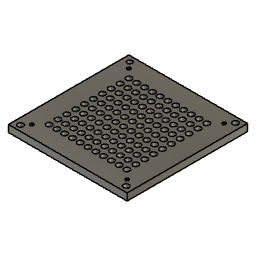
WC_Zwischenboden (Autodesk Fusion 360 design; units mm, degrees)
Autodesk Fusion 360 part; units mm, degrees
note: some values were not read from the file. Set by a fixed rule: which face or edge a step refers to.
(part 1 of 3)
sketch "Skizze1" plane through (0, 0, 0) normal (0, 0, 1) x (1, 0, 0)
  line L0 (0.1074, 0.221) -> (507.9074, 0.221)
  line L1 (507.9074, 0.221) -> (507.9074, -514.979)
  line L2 (507.9074, -514.979) -> (0.1074, -514.979)
  line L3 (0.1074, -514.979) -> (0.1074, 0.221)
  circle A0 centre (87.5074, -86.379) radius 12
  circle A1 centre (28.1074, -23.779) radius 10.8095
  circle A2 centre (479.9074, -23.779) radius 12
  circle A3 centre (120.8074, -86.379) radius 12
  circle A4 centre (154.1074, -86.379) radius 12
  circle A5 centre (187.4074, -86.379) radius 12
  circle A6 centre (220.7074, -86.379) radius 12
  circle A7 centre (254.0074, -86.379) radius 12
  circle A8 centre (287.3074, -86.379) radius 12
  circle A9 centre (320.6074, -86.379) radius 12
  circle A10 centre (353.9074, -86.379) radius 12
  circle A11 centre (387.2074, -86.379) radius 12
  circle A12 centre (420.5074, -86.379) radius 12
  circle A13 centre (87.5074, -124.379) radius 12
  circle A14 centre (120.8074, -124.379) radius 12
  circle A15 centre (154.1074, -124.379) radius 12
  circle A16 centre (187.4074, -124.379) radius 12
  circle A17 centre (220.7074, -124.379) radius 12
  circle A18 centre (254.0074, -124.379) radius 12
  circle A19 centre (287.3074, -124.379) radius 12
  circle A20 centre (320.6074, -124.379) radius 12
  circle A21 centre (353.9074, -124.379) radius 12
  circle A22 centre (387.2074, -124.379) radius 12
  circle A23 centre (420.5074, -124.379) radius 12
  circle A24 centre (87.5074, -162.379) radius 12
  circle A25 centre (120.8074, -162.379) radius 12
  circle A26 centre (154.1074, -162.379) radius 12
  circle A27 centre (187.4074, -162.379) radius 12
  circle A28 centre (220.7074, -162.379) radius 12
  circle A29 centre (254.0074, -162.379) radius 12
  circle A30 centre (287.3074, -162.379) radius 12
  circle A31 centre (320.6074, -162.379) radius 12
  circle A32 centre (353.9074, -162.379) radius 12
  circle A33 centre (387.2074, -162.379) radius 12
  circle A34 centre (420.5074, -162.379) radius 12
  circle A35 centre (87.5074, -200.379) radius 12
  circle A36 centre (120.8074, -200.379) radius 12
  circle A37 centre (154.1074, -200.379) radius 12
  circle A38 centre (187.4074, -200.379) radius 12
  circle A39 centre (220.7074, -200.379) radius 12
  circle A40 centre (254.0074, -200.379) radius 12
  circle A41 centre (287.3074, -200.379) radius 12
  circle A42 centre (320.6074, -200.379) radius 12
  circle A43 centre (353.9074, -200.379) radius 12
  circle A44 centre (387.2074, -200.379) radius 12
  circle A45 centre (420.5074, -200.379) radius 12
  circle A46 centre (87.5074, -238.379) radius 12
  circle A47 centre (120.8074, -238.379) radius 12
  circle A48 centre (154.1074, -238.379) radius 12
  circle A49 centre (187.4074, -238.379) radius 12
  circle A50 centre (220.7074, -238.379) radius 12
  circle A51 centre (254.0074, -238.379) radius 12
  circle A52 centre (287.3074, -238.379) radius 12
  circle A53 centre (320.6074, -238.379) radius 12
  circle A54 centre (353.9074, -238.379) radius 12
  circle A55 centre (387.2074, -238.379) radius 12
  circle A56 centre (420.5074, -238.379) radius 12
  circle A57 centre (87.5074, -276.379) radius 12
  circle A58 centre (120.8074, -276.379) radius 12
  circle A59 centre (154.1074, -276.379) radius 12
  circle A60 centre (187.4074, -276.379) radius 12
  circle A61 centre (220.7074, -276.379) radius 12
  circle A62 centre (254.0074, -276.379) radius 12
  circle A63 centre (287.3074, -276.379) radius 12
  circle A64 centre (320.6074, -276.379) radius 12
  circle A65 centre (353.9074, -276.379) radius 12
  circle A66 centre (387.2074, -276.379) radius 12
  circle A67 centre (420.5074, -276.379) radius 12
  circle A68 centre (87.5074, -314.379) radius 12
  circle A69 centre (120.8074, -314.379) radius 12
  circle A70 centre (154.1074, -314.379) radius 12
  circle A71 centre (187.4074, -314.379) radius 12
  circle A72 centre (220.7074, -314.379) radius 12
  circle A73 centre (254.0074, -314.379) radius 12
  circle A74 centre (287.3074, -314.379) radius 12
  circle A75 centre (320.6074, -314.379) radius 12
  circle A76 centre (353.9074, -314.379) radius 12
  circle A77 centre (387.2074, -314.379) radius 12
  circle A78 centre (420.5074, -314.379) radius 12
  circle A79 centre (87.5074, -352.379) radius 12
  circle A80 centre (120.8074, -352.379) radius 12
  circle A81 centre (154.1074, -352.379) radius 12
  circle A82 centre (187.4074, -352.379) radius 12
  circle A83 centre (220.7074, -352.379) radius 12
  circle A84 centre (254.0074, -352.379) radius 12
  circle A85 centre (287.3074, -352.379) radius 12
  circle A86 centre (320.6074, -352.379) radius 12
  circle A87 centre (353.9074, -352.379) radius 12
  circle A88 centre (387.2074, -352.379) radius 12
  circle A89 centre (420.5074, -352.379) radius 12
  circle A90 centre (87.5074, -390.379) radius 12
  circle A91 centre (120.8074, -390.379) radius 12
  circle A92 centre (154.1074, -390.379) radius 12
  circle A93 centre (187.4074, -390.379) radius 12
  circle A94 centre (220.7074, -390.379) radius 12
  circle A95 centre (254.0074, -390.379) radius 12
  circle A96 centre (287.3074, -390.379) radius 12
  circle A97 centre (320.6074, -390.379) radius 12
  circle A98 centre (353.9074, -390.379) radius 12
  circle A99 centre (387.2074, -390.379) radius 12
  circle A100 centre (420.5074, -390.379) radius 12
  circle A101 centre (87.5074, -428.379) radius 12
  circle A102 centre (120.8074, -428.379) radius 12
  circle A103 centre (154.1074, -428.379) radius 12
  circle A104 centre (187.4074, -428.379) radius 12
  circle A105 centre (220.7074, -428.379) radius 12
  circle A106 centre (254.0074, -428.379) radius 12
  circle A107 centre (287.3074, -428.379) radius 12
  circle A108 centre (320.6074, -428.379) radius 12
  circle A109 centre (353.9074, -428.379) radius 12
  circle A110 centre (387.2074, -428.379) radius 12
  circle A111 centre (420.5074, -428.379) radius 12
  circle A112 centre (28.1074, -490.979) radius 12
  circle A113 centre (479.9074, -490.979) radius 12
  dimension "d1" = 24
  dimension "d2" = 87.4
  dimension "d3" = 86.6
  dimension "d6" = 21.619
  dimension "d7" = 28
  dimension "d8" = 24
  dimension "d38" = 24
  dimension "d39" = 24
  dimension "d40" = 28
  dimension "d131" = 33.3
  dimension "d132" = -38
  dimension "d133" = 38
  dimension "d134" = 38
  dimension "d135" = 38
  dimension "d136" = 38
  dimension "d137" = 38
  dimension "d138" = 38
  dimension "d139" = 38
  dimension "d140" = 38
  dimension "d141" = 38
  dimension "d142" = 86.6
  dimension "d143" = 33.3
  dimension "d144" = 33.3
  dimension "d145" = 33.3
  dimension "d146" = 33.3
  dimension "d147" = 33.3
  dimension "d148" = 33.3
  dimension "d149" = 33.3
  dimension "d150" = 33.3
  dimension "d151" = 33.3
  dimension "d152" = 33.3
  dimension "d153" = 87.4
  dimension "d154" = 24
  dimension "d155" = 28
  dimension "d156" = 24
  dimension "d157" = 24
  dimension "d158" = 24
  dimension "d159" = 28
  constraint horizontal L0
  constraint vertical L1
  constraint vertical L3
  measures "d1" diameter of A0
  measures "d2" distance of L3 A0.centre
  measures "d3" distance of L0 A0.centre
  measures "d6" diameter of A1
  measures "d7" distance of L3 A1.centre
  measures "d8" distance of L0 A1.centre
  measures "d38" diameter of A2
  measures "d39" distance of L0 A2.centre
  measures "d40" distance of L1 A2.centre
  measures "d133" distance of A0.centre A13.centre
  measures "d134" distance of A13.centre A24.centre
  measures "d135" distance of A24.centre A35.centre
  measures "d136" distance of A35.centre A46.centre
  measures "d137" distance of A46.centre A57.centre
  measures "d138" distance of A57.centre A68.centre
  measures "d139" distance of A68.centre A79.centre
  measures "d140" distance of A79.centre A90.centre
  measures "d141" distance of A90.centre A101.centre
  measures "d142" distance of L2 A101.centre
  measures "d143" distance of A0.centre A3.centre
  measures "d144" distance of A3.centre A4.centre
  measures "d145" distance of A4.centre A5.centre
  measures "d146" distance of A5.centre A6.centre
  measures "d147" distance of A6.centre A7.centre
  measures "d148" distance of A7.centre A8.centre
  measures "d149" distance of A8.centre A9.centre
  measures "d150" distance of A9.centre A10.centre
  measures "d151" distance of A10.centre A11.centre
  measures "d152" distance of A11.centre A12.centre
  measures "d153" distance of L1 A12.centre
  measures "d154" diameter of A112
  measures "d155" distance of L3 A112.centre
  measures "d156" distance of L2 A112.centre
  measures "d157" diameter of A113
  measures "d158" distance of L2 A113.centre
  measures "d159" distance of L1 A113.centre
extrude "Extrusion1" add sketch "Skizze1" along normal blind 20
sketch "Skizze2" plane through (0, 0, 20) normal (0, 0, 1) x (-1, 0, 0)
  circle A0 centre (-387.2074, 124.379) radius 12
  circle A1 centre (-353.9074, 124.379) radius 12
  circle A2 centre (-320.6074, 124.379) radius 12
  circle A3 centre (-287.3074, 124.379) radius 12
  circle A4 centre (-254.0074, 124.379) radius 12
  circle A5 centre (-220.7074, 124.379) radius 12
  circle A6 centre (-187.4074, 124.379) radius 12
  circle A7 centre (-154.1074, 124.379) radius 12
  circle A8 centre (-120.8074, 124.379) radius 12
  circle A9 centre (-87.5074, 124.379) radius 12
  circle A10 centre (-420.5074, 86.379) radius 12
  circle A11 centre (-387.2074, 86.379) radius 12
  circle A12 centre (-353.9074, 86.379) radius 12
  circle A13 centre (-320.6074, 86.379) radius 12
  circle A14 centre (-287.3074, 86.379) radius 12
  circle A15 centre (-254.0074, 86.379) radius 12
  circle A16 centre (-220.7074, 86.379) radius 12
  circle A17 centre (-187.4074, 86.379) radius 12
  circle A18 centre (-154.1074, 86.379) radius 12
  circle A19 centre (-120.8074, 86.379) radius 12
  circle A20 centre (-479.9074, 23.779) radius 12
  circle A21 centre (-28.1074, 23.779) radius 10.8095
  circle A22 centre (-87.5074, 86.379) radius 12
  circle A23 centre (-387.2074, 238.379) radius 12
  circle A24 centre (-420.5074, 238.379) radius 12
  circle A25 centre (-87.5074, 276.379) radius 12
  circle A26 centre (-120.8074, 276.379) radius 12
  circle A27 centre (-154.1074, 276.379) radius 12
  circle A28 centre (-187.4074, 276.379) radius 12
  circle A29 centre (-220.7074, 276.379) radius 12
  circle A30 centre (-254.0074, 276.379) radius 12
  circle A31 centre (-287.3074, 276.379) radius 12
  circle A32 centre (-320.6074, 276.379) radius 12
  circle A33 centre (-353.9074, 276.379) radius 12
  circle A34 centre (-387.2074, 276.379) radius 12
  circle A35 centre (-420.5074, 276.379) radius 12
  circle A36 centre (-87.5074, 314.379) radius 12
  circle A37 centre (-120.8074, 314.379) radius 12
  circle A38 centre (-154.1074, 314.379) radius 12
  circle A39 centre (-187.4074, 314.379) radius 12
  circle A40 centre (-220.7074, 314.379) radius 12
  circle A41 centre (-254.0074, 314.379) radius 12
  circle A42 centre (-287.3074, 314.379) radius 12
  circle A43 centre (-320.6074, 314.379) radius 12
  circle A44 centre (-353.9074, 314.379) radius 12
  circle A45 centre (-387.2074, 314.379) radius 12
  circle A46 centre (-420.5074, 314.379) radius 12
  circle A47 centre (-87.5074, 352.379) radius 12
  circle A48 centre (-120.8074, 352.379) radius 12
  circle A49 centre (-154.1074, 352.379) radius 12
  circle A50 centre (-187.4074, 352.379) radius 12
  circle A51 centre (-220.7074, 352.379) radius 12
  circle A52 centre (-254.0074, 352.379) radius 12
  circle A53 centre (-353.9074, 238.379) radius 12
  circle A54 centre (-320.6074, 238.379) radius 12
  circle A55 centre (-287.3074, 238.379) radius 12
  circle A56 centre (-254.0074, 238.379) radius 12
  circle A57 centre (-220.7074, 238.379) radius 12
  circle A58 centre (-187.4074, 238.379) radius 12
  circle A59 centre (-154.1074, 238.379) radius 12
  circle A60 centre (-120.8074, 238.379) radius 12
  circle A61 centre (-87.5074, 238.379) radius 12
  circle A62 centre (-420.5074, 200.379) radius 12
  circle A63 centre (-387.2074, 200.379) radius 12
  circle A64 centre (-353.9074, 200.379) radius 12
  circle A65 centre (-320.6074, 200.379) radius 12
  circle A66 centre (-287.3074, 200.379) radius 12
  circle A67 centre (-254.0074, 200.379) radius 12
  circle A68 centre (-220.7074, 200.379) radius 12
  circle A69 centre (-187.4074, 200.379) radius 12
  circle A70 centre (-154.1074, 200.379) radius 12
  circle A71 centre (-120.8074, 200.379) radius 12
  circle A72 centre (-87.5074, 200.379) radius 12
  circle A73 centre (-420.5074, 162.379) radius 12
  circle A74 centre (-387.2074, 162.379) radius 12
  circle A75 centre (-353.9074, 162.379) radius 12
  circle A76 centre (-320.6074, 162.379) radius 12
  circle A77 centre (-287.3074, 162.379) radius 12
  circle A78 centre (-254.0074, 162.379) radius 12
  circle A79 centre (-220.7074, 162.379) radius 12
  circle A80 centre (-187.4074, 162.379) radius 12
  circle A81 centre (-154.1074, 162.379) radius 12
  circle A82 centre (-120.8074, 162.379) radius 12
  circle A83 centre (-87.5074, 162.379) radius 12
  circle A84 centre (-420.5074, 124.379) radius 12
  circle A85 centre (-320.6074, 352.379) radius 12
  circle A86 centre (-353.9074, 352.379) radius 12
  circle A87 centre (-387.2074, 352.379) radius 12
  circle A88 centre (-420.5074, 352.379) radius 12
  circle A89 centre (-87.5074, 390.379) radius 12
  circle A90 centre (-120.8074, 390.379) radius 12
  circle A91 centre (-154.1074, 390.379) radius 12
  circle A92 centre (-187.4074, 390.379) radius 12
  circle A93 centre (-220.7074, 390.379) radius 12
  circle A94 centre (-254.0074, 390.379) radius 12
  circle A95 centre (-287.3074, 390.379) radius 12
  circle A96 centre (-320.6074, 390.379) radius 12
  circle A97 centre (-353.9074, 390.379) radius 12
  circle A98 centre (-387.2074, 390.379) radius 12
  circle A99 centre (-420.5074, 390.379) radius 12
  circle A100 centre (-87.5074, 428.379) radius 12
  circle A101 centre (-120.8074, 428.379) radius 12
  circle A102 centre (-154.1074, 428.379) radius 12
  circle A103 centre (-187.4074, 428.379) radius 12
  circle A104 centre (-220.7074, 428.379) radius 12
  circle A105 centre (-254.0074, 428.379) radius 12
  circle A106 centre (-287.3074, 428.379) radius 12
  circle A107 centre (-320.6074, 428.379) radius 12
  circle A108 centre (-353.9074, 428.379) radius 12
  circle A109 centre (-387.2074, 428.379) radius 12
  circle A110 centre (-420.5074, 428.379) radius 12
  circle A111 centre (-28.1074, 490.979) radius 12
  circle A112 centre (-479.9074, 490.979) radius 12
  circle A113 centre (-287.3074, 352.379) radius 12
  line L0 (-0.1074, 514.979) -> (-507.9074, 514.979)
  line L1 (-507.9074, 514.979) -> (-507.9074, -0.221)
  line L2 (-507.9074, -0.221) -> (-0.1074, -0.221)
  line L3 (-0.1074, -0.221) -> (-0.1074, 514.979)
extrude "Extrusion2" add sketch "Skizze2" along normal blind 10
sketch "Skizze4" plane through (0, 0, 0) normal (0, 0, -1) x (1, 0, 0)
  circle A0 centre (387.2074, 124.379) radius 12
  circle A1 centre (353.9074, 124.379) radius 12
  circle A2 centre (320.6074, 124.379) radius 12
  circle A3 centre (287.3074, 124.379) radius 12
  circle A4 centre (254.0074, 124.379) radius 12
  circle A5 centre (220.7074, 124.379) radius 12
  circle A6 centre (187.4074, 124.379) radius 12
  circle A7 centre (154.1074, 124.379) radius 12
  circle A8 centre (120.8074, 124.379) radius 12
  circle A9 centre (87.5074, 124.379) radius 12
  circle A10 centre (420.5074, 86.379) radius 12
  circle A11 centre (387.2074, 86.379) radius 12
  circle A12 centre (353.9074, 86.379) radius 12
  circle A13 centre (320.6074, 86.379) radius 12
  circle A14 centre (287.3074, 86.379) radius 12
  circle A15 centre (254.0074, 86.379) radius 12
  circle A16 centre (220.7074, 86.379) radius 12
  circle A17 centre (187.4074, 86.379) radius 12
  circle A18 centre (154.1074, 86.379) radius 12
  circle A19 centre (120.8074, 86.379) radius 12
  circle A20 centre (479.9074, 23.779) radius 12
  circle A21 centre (28.1074, 23.779) radius 10.8095
  circle A22 centre (87.5074, 86.379) radius 12
  circle A23 centre (387.2074, 238.379) radius 12
  circle A24 centre (420.5074, 238.379) radius 12
  circle A25 centre (87.5074, 276.379) radius 12
  circle A26 centre (120.8074, 276.379) radius 12
  circle A27 centre (154.1074, 276.379) radius 12
  circle A28 centre (187.4074, 276.379) radius 12
  circle A29 centre (220.7074, 276.379) radius 12
  circle A30 centre (254.0074, 276.379) radius 12
  circle A31 centre (287.3074, 276.379) radius 12
  circle A32 centre (320.6074, 276.379) radius 12
  circle A33 centre (353.9074, 276.379) radius 12
  circle A34 centre (387.2074, 276.379) radius 12
  circle A35 centre (420.5074, 276.379) radius 12
  circle A36 centre (87.5074, 314.379) radius 12
  circle A37 centre (120.8074, 314.379) radius 12
  circle A38 centre (154.1074, 314.379) radius 12
  circle A39 centre (187.4074, 314.379) radius 12
  circle A40 centre (220.7074, 314.379) radius 12
  circle A41 centre (254.0074, 314.379) radius 12
  circle A42 centre (287.3074, 314.379) radius 12
  circle A43 centre (320.6074, 314.379) radius 12
  circle A44 centre (353.9074, 314.379) radius 12
  circle A45 centre (387.2074, 314.379) radius 12
  circle A46 centre (420.5074, 314.379) radius 12
  circle A47 centre (87.5074, 352.379) radius 12
  circle A48 centre (120.8074, 352.379) radius 12
  circle A49 centre (154.1074, 352.379) radius 12
  circle A50 centre (187.4074, 352.379) radius 12
  circle A51 centre (220.7074, 352.379) radius 12
  circle A52 centre (254.0074, 352.379) radius 12
  circle A53 centre (353.9074, 238.379) radius 12
  circle A54 centre (320.6074, 238.379) radius 12
  circle A55 centre (287.3074, 238.379) radius 12
  circle A56 centre (254.0074, 238.379) radius 12
  circle A57 centre (220.7074, 238.379) radius 12
  circle A58 centre (187.4074, 238.379) radius 12
  circle A59 centre (154.1074, 238.379) radius 12
  circle A60 centre (120.8074, 238.379) radius 12
  circle A61 centre (87.5074, 238.379) radius 12
  circle A62 centre (420.5074, 200.379) radius 12
  circle A63 centre (387.2074, 200.379) radius 12
  circle A64 centre (353.9074, 200.379) radius 12
  circle A65 centre (320.6074, 200.379) radius 12
  circle A66 centre (287.3074, 200.379) radius 12
  circle A67 centre (254.0074, 200.379) radius 12
  circle A68 centre (220.7074, 200.379) radius 12
  circle A69 centre (187.4074, 200.379) radius 12
  circle A70 centre (154.1074, 200.379) radius 12
  circle A71 centre (120.8074, 200.379) radius 12
  circle A72 centre (87.5074, 200.379) radius 12
  circle A73 centre (420.5074, 162.379) radius 12
  circle A74 centre (387.2074, 162.379) radius 12
  circle A75 centre (353.9074, 162.379) radius 12
  circle A76 centre (320.6074, 162.379) radius 12
  circle A77 centre (287.3074, 162.379) radius 12
  circle A78 centre (254.0074, 162.379) radius 12
  circle A79 centre (220.7074, 162.379) radius 12
  circle A80 centre (187.4074, 162.379) radius 12
  circle A81 centre (154.1074, 162.379) radius 12
  circle A82 centre (120.8074, 162.379) radius 12
  circle A83 centre (87.5074, 162.379) radius 12
  circle A84 centre (420.5074, 124.379) radius 12
  circle A85 centre (320.6074, 352.379) radius 12
  circle A86 centre (353.9074, 352.379) radius 12
  circle A87 centre (387.2074, 352.379) radius 12
  circle A88 centre (420.5074, 352.379) radius 12
  circle A89 centre (87.5074, 390.379) radius 12
  circle A90 centre (120.8074, 390.379) radius 12
  circle A91 centre (154.1074, 390.379) radius 12
  circle A92 centre (187.4074, 390.379) radius 12
  circle A93 centre (220.7074, 390.379) radius 12
  circle A94 centre (254.0074, 390.379) radius 12
  circle A95 centre (287.3074, 390.379) radius 12
  circle A96 centre (320.6074, 390.379) radius 12
  circle A97 centre (353.9074, 390.379) radius 12
  circle A98 centre (387.2074, 390.379) radius 12
  circle A99 centre (420.5074, 390.379) radius 12
  circle A100 centre (87.5074, 428.379) radius 12
  circle A101 centre (120.8074, 428.379) radius 12
  circle A102 centre (154.1074, 428.379) radius 12
  circle A103 centre (187.4074, 428.379) radius 12
  circle A104 centre (220.7074, 428.379) radius 12
  circle A105 centre (254.0074, 428.379) radius 12
  circle A106 centre (287.3074, 428.379) radius 12
  circle A107 centre (320.6074, 428.379) radius 12
  circle A108 centre (353.9074, 428.379) radius 12
  circle A109 centre (387.2074, 428.379) radius 12
  circle A110 centre (420.5074, 428.379) radius 12
  circle A111 centre (28.1074, 490.979) radius 12
  circle A112 centre (479.9074, 490.979) radius 12
  circle A113 centre (287.3074, 352.379) radius 12
  line L0 (507.9074, 514.979) -> (0.1074, 514.979)
  line L1 (0.1074, 514.979) -> (0.1074, -0.221)
  line L2 (0.1074, -0.221) -> (507.9074, -0.221)
  line L3 (507.9074, -0.221) -> (507.9074, 514.979)
  line L4 (10.1074, 464.979) -> (60.1074, 464.979)
  line L5 (60.1074, 464.979) -> (60.1074, 49.779)
  line L6 (60.1074, 49.779) -> (10.1074, 49.779)
  line L7 (10.1074, 49.779) -> (10.1074, 464.979)
  dimension "d180" = 50
  dimension "d181" = 50
  dimension "d182" = 10
  dimension "d183" = 50
  constraint horizontal L4
  constraint vertical L5
  constraint horizontal L6
  constraint vertical L7
  measures "d180" distance of L0 L4
  measures "d181" distance of L2 L6
  measures "d182" distance of L1 L7
  measures "d183" distance of L5 L7
extrude "Extrusion3" cut sketch "Skizze4" against normal blind 20 contours L4 L5 L6 L7
sketch "Skizze5" plane through (0, 0, 0) normal (0, 0, -1) x (1, 0, 0)
  line L0 (60.1074, 464.979) -> (60.1074, 49.779)
  line L1 (60.1074, 49.779) -> (10.1074, 49.779)
  line L2 (10.1074, 49.779) -> (10.1074, 464.979)
  line L3 (10.1074, 464.979) -> (60.1074, 464.979)
  circle A0 centre (387.2074, 124.379) radius 12
  circle A1 centre (353.9074, 124.379) radius 12
  circle A2 centre (320.6074, 124.379) radius 12
  circle A3 centre (287.3074, 124.379) radius 12
  circle A4 centre (254.0074, 124.379) radius 12
  circle A5 centre (220.7074, 124.379) radius 12
  circle A6 centre (187.4074, 124.379) radius 12
  circle A7 centre (154.1074, 124.379) radius 12
  circle A8 centre (120.8074, 124.379) radius 12
  circle A9 centre (87.5074, 124.379) radius 12
  circle A10 centre (420.5074, 86.379) radius 12
  circle A11 centre (387.2074, 86.379) radius 12
  circle A12 centre (353.9074, 86.379) radius 12
  circle A13 centre (320.6074, 86.379) radius 12
  circle A14 centre (287.3074, 86.379) radius 12
  circle A15 centre (254.0074, 86.379) radius 12
  circle A16 centre (220.7074, 86.379) radius 12
  circle A17 centre (187.4074, 86.379) radius 12
  circle A18 centre (154.1074, 86.379) radius 12
  circle A19 centre (120.8074, 86.379) radius 12
  circle A20 centre (479.9074, 23.779) radius 12
  circle A21 centre (28.1074, 23.779) radius 10.8095
  circle A22 centre (87.5074, 86.379) radius 12
  circle A23 centre (387.2074, 238.379) radius 12
  circle A24 centre (420.5074, 238.379) radius 12
  circle A25 centre (87.5074, 276.379) radius 12
  circle A26 centre (120.8074, 276.379) radius 12
  circle A27 centre (154.1074, 276.379) radius 12
  circle A28 centre (187.4074, 276.379) radius 12
  circle A29 centre (220.7074, 276.379) radius 12
  circle A30 centre (254.0074, 276.379) radius 12
  circle A31 centre (287.3074, 276.379) radius 12
  circle A32 centre (320.6074, 276.379) radius 12
  circle A33 centre (353.9074, 276.379) radius 12
  circle A34 centre (387.2074, 276.379) radius 12
  circle A35 centre (420.5074, 276.379) radius 12
  circle A36 centre (87.5074, 314.379) radius 12
  circle A37 centre (120.8074, 314.379) radius 12
  circle A38 centre (154.1074, 314.379) radius 12
  circle A39 centre (187.4074, 314.379) radius 12
  circle A40 centre (220.7074, 314.379) radius 12
  circle A41 centre (254.0074, 314.379) radius 12
  circle A42 centre (287.3074, 314.379) radius 12
  circle A43 centre (320.6074, 314.379) radius 12
  circle A44 centre (353.9074, 314.379) radius 12
  circle A45 centre (387.2074, 314.379) radius 12
  circle A46 centre (420.5074, 314.379) radius 12
  circle A47 centre (87.5074, 352.379) radius 12
  circle A48 centre (120.8074, 352.379) radius 12
  circle A49 centre (154.1074, 352.379) radius 12
  circle A50 centre (187.4074, 352.379) radius 12
  circle A51 centre (220.7074, 352.379) radius 12
  circle A52 centre (254.0074, 352.379) radius 12
  circle A53 centre (353.9074, 238.379) radius 12
  circle A54 centre (320.6074, 238.379) radius 12
  circle A55 centre (287.3074, 238.379) radius 12
  circle A56 centre (254.0074, 238.379) radius 12
  circle A57 centre (220.7074, 238.379) radius 12
  circle A58 centre (187.4074, 238.379) radius 12
  circle A59 centre (154.1074, 238.379) radius 12
  circle A60 centre (120.8074, 238.379) radius 12
  circle A61 centre (87.5074, 238.379) radius 12
  circle A62 centre (420.5074, 200.379) radius 12
  circle A63 centre (387.2074, 200.379) radius 12
  circle A64 centre (353.9074, 200.379) radius 12
  circle A65 centre (320.6074, 200.379) radius 12
  circle A66 centre (287.3074, 200.379) radius 12
  circle A67 centre (254.0074, 200.379) radius 12
  circle A68 centre (220.7074, 200.379) radius 12
  circle A69 centre (187.4074, 200.379) radius 12
  circle A70 centre (154.1074, 200.379) radius 12
  circle A71 centre (120.8074, 200.379) radius 12
  circle A72 centre (87.5074, 200.379) radius 12
  circle A73 centre (420.5074, 162.379) radius 12
  circle A74 centre (387.2074, 162.379) radius 12
  circle A75 centre (353.9074, 162.379) radius 12
  circle A76 centre (320.6074, 162.379) radius 12
  circle A77 centre (287.3074, 162.379) radius 12
  circle A78 centre (254.0074, 162.379) radius 12
  circle A79 centre (220.7074, 162.379) radius 12
  circle A80 centre (187.4074, 162.379) radius 12
  circle A81 centre (154.1074, 162.379) radius 12
  circle A82 centre (120.8074, 162.379) radius 12
  circle A83 centre (87.5074, 162.379) radius 12
  circle A84 centre (420.5074, 124.379) radius 12
  circle A85 centre (320.6074, 352.379) radius 12
  circle A86 centre (353.9074, 352.379) radius 12
  circle A87 centre (387.2074, 352.379) radius 12
  circle A88 centre (420.5074, 352.379) radius 12
  circle A89 centre (87.5074, 390.379) radius 12
  circle A90 centre (120.8074, 390.379) radius 12
  circle A91 centre (154.1074, 390.379) radius 12
  circle A92 centre (187.4074, 390.379) radius 12
  circle A93 centre (220.7074, 390.379) radius 12
  circle A94 centre (254.0074, 390.379) radius 12
  circle A95 centre (287.3074, 390.379) radius 12
  circle A96 centre (320.6074, 390.379) radius 12
  circle A97 centre (353.9074, 390.379) radius 12
  circle A98 centre (387.2074, 390.379) radius 12
  circle A99 centre (420.5074, 390.379) radius 12
  circle A100 centre (87.5074, 428.379) radius 12
  circle A101 centre (120.8074, 428.379) radius 12
  circle A102 centre (154.1074, 428.379) radius 12
  circle A103 centre (187.4074, 428.379) radius 12
  circle A104 centre (220.7074, 428.379) radius 12
  circle A105 centre (254.0074, 428.379) radius 12
  circle A106 centre (287.3074, 428.379) radius 12
  circle A107 centre (320.6074, 428.379) radius 12
  circle A108 centre (353.9074, 428.379) radius 12
  circle A109 centre (387.2074, 428.379) radius 12
  circle A110 centre (420.5074, 428.379) radius 12
  circle A111 centre (28.1074, 490.979) radius 12
  circle A112 centre (479.9074, 490.979) radius 12
  circle A113 centre (287.3074, 352.379) radius 12
  line L4 (507.9074, 514.979) -> (0.1074, 514.979)
  line L5 (0.1074, 514.979) -> (0.1074, -0.221)
  line L6 (0.1074, -0.221) -> (507.9074, -0.221)
  line L7 (507.9074, -0.221) -> (507.9074, 514.979)
  line L8 (50.1074, 504.979) -> (457.9074, 504.979)
  line L9 (457.9074, 504.979) -> (457.9074, 449.979)
  line L10 (457.9074, 449.979) -> (50.1074, 449.979)
  line L11 (50.1074, 449.979) -> (50.1074, 504.979)
  dimension "d186" = 50
  dimension "d187" = 50
  dimension "d188" = 10
  dimension "d189" = 55
  constraint horizontal L8
  constraint vertical L9
  constraint horizontal L10
  constraint vertical L11
  measures "d186" distance of L5 L11
  measures "d187" distance of L7 L9
  measures "d188" distance of L4 L8
  measures "d189" distance of L8 L10
extrude "Extrusion4" cut sketch "Skizze5" against normal blind 20 contours L0 L3 L8 L9 L10 L11
sketch "Skizze6" plane through (0, 0, 0) normal (0, 0, -1) x (1, 0, 0)
  line L0 (457.9074, 449.979) -> (60.1074, 449.979)
  line L1 (60.1074, 449.979) -> (60.1074, 49.779)
  line L2 (60.1074, 49.779) -> (10.1074, 49.779)
  line L3 (10.1074, 49.779) -> (10.1074, 464.979)
  line L4 (10.1074, 464.979) -> (50.1074, 464.979)
  line L5 (50.1074, 464.979) -> (50.1074, 504.979)
  line L6 (50.1074, 504.979) -> (457.9074, 504.979)
  line L7 (457.9074, 504.979) -> (457.9074, 449.979)
  circle A0 centre (387.2074, 124.379) radius 12
  circle A1 centre (353.9074, 124.379) radius 12
  circle A2 centre (320.6074, 124.379) radius 12
  circle A3 centre (287.3074, 124.379) radius 12
  circle A4 centre (254.0074, 124.379) radius 12
  circle A5 centre (220.7074, 124.379) radius 12
  circle A6 centre (187.4074, 124.379) radius 12
  circle A7 centre (154.1074, 124.379) radius 12
  circle A8 centre (120.8074, 124.379) radius 12
  circle A9 centre (87.5074, 124.379) radius 12
  circle A10 centre (420.5074, 86.379) radius 12
  circle A11 centre (387.2074, 86.379) radius 12
  circle A12 centre (353.9074, 86.379) radius 12
  circle A13 centre (320.6074, 86.379) radius 12
  circle A14 centre (287.3074, 86.379) radius 12
  circle A15 centre (254.0074, 86.379) radius 12
  circle A16 centre (220.7074, 86.379) radius 12
  circle A17 centre (187.4074, 86.379) radius 12
  circle A18 centre (154.1074, 86.379) radius 12
  circle A19 centre (120.8074, 86.379) radius 12
  circle A20 centre (479.9074, 23.779) radius 12
  circle A21 centre (28.1074, 23.779) radius 10.8095
  circle A22 centre (87.5074, 86.379) radius 12
  circle A23 centre (387.2074, 238.379) radius 12
  circle A24 centre (420.5074, 238.379) radius 12
  circle A25 centre (87.5074, 276.379) radius 12
  circle A26 centre (120.8074, 276.379) radius 12
  circle A27 centre (154.1074, 276.379) radius 12
  circle A28 centre (187.4074, 276.379) radius 12
  circle A29 centre (220.7074, 276.379) radius 12
  circle A30 centre (254.0074, 276.379) radius 12
  circle A31 centre (287.3074, 276.379) radius 12
  circle A32 centre (320.6074, 276.379) radius 12
  circle A33 centre (353.9074, 276.379) radius 12
  circle A34 centre (387.2074, 276.379) radius 12
  circle A35 centre (420.5074, 276.379) radius 12
  circle A36 centre (87.5074, 314.379) radius 12
  circle A37 centre (120.8074, 314.379) radius 12
  circle A38 centre (154.1074, 314.379) radius 12
  circle A39 centre (187.4074, 314.379) radius 12
  circle A40 centre (220.7074, 314.379) radius 12
  circle A41 centre (254.0074, 314.379) radius 12
  circle A42 centre (287.3074, 314.379) radius 12
  circle A43 centre (320.6074, 314.379) radius 12
  circle A44 centre (353.9074, 314.379) radius 12
  circle A45 centre (387.2074, 314.379) radius 12
  circle A46 centre (420.5074, 314.379) radius 12
  circle A47 centre (87.5074, 352.379) radius 12
  circle A48 centre (120.8074, 352.379) radius 12
  circle A49 centre (154.1074, 352.379) radius 12
  circle A50 centre (187.4074, 352.379) radius 12
  circle A51 centre (220.7074, 352.379) radius 12
  circle A52 centre (254.0074, 352.379) radius 12
  circle A53 centre (353.9074, 238.379) radius 12
  circle A54 centre (320.6074, 238.379) radius 12
  circle A55 centre (287.3074, 238.379) radius 12
  circle A56 centre (254.0074, 238.379) radius 12
  circle A57 centre (220.7074, 238.379) radius 12
  circle A58 centre (187.4074, 238.379) radius 12
  circle A59 centre (154.1074, 238.379) radius 12
  circle A60 centre (120.8074, 238.379) radius 12
  circle A61 centre (87.5074, 238.379) radius 12
  circle A62 centre (420.5074, 200.379) radius 12
  circle A63 centre (387.2074, 200.379) radius 12
  circle A64 centre (353.9074, 200.379) radius 12
  circle A65 centre (320.6074, 200.379) radius 12
  circle A66 centre (287.3074, 200.379) radius 12
  circle A67 centre (254.0074, 200.379) radius 12
  circle A68 centre (220.7074, 200.379) radius 12
  circle A69 centre (187.4074, 200.379) radius 12
  circle A70 centre (154.1074, 200.379) radius 12
  circle A71 centre (120.8074, 200.379) radius 12
  circle A72 centre (87.5074, 200.379) radius 12
  circle A73 centre (420.5074, 162.379) radius 12
  circle A74 centre (387.2074, 162.379) radius 12
  circle A75 centre (353.9074, 162.379) radius 12
  circle A76 centre (320.6074, 162.379) radius 12
  circle A77 centre (287.3074, 162.379) radius 12
  circle A78 centre (254.0074, 162.379) radius 12
  circle A79 centre (220.7074, 162.379) radius 12
  circle A80 centre (187.4074, 162.379) radius 12
  circle A81 centre (154.1074, 162.379) radius 12
  circle A82 centre (120.8074, 162.379) radius 12
  circle A83 centre (87.5074, 162.379) radius 12
  circle A84 centre (420.5074, 124.379) radius 12
  circle A85 centre (320.6074, 352.379) radius 12
  circle A86 centre (353.9074, 352.379) radius 12
  circle A87 centre (387.2074, 352.379) radius 12
  circle A88 centre (420.5074, 352.379) radius 12
  circle A89 centre (87.5074, 390.379) radius 12
  circle A90 centre (120.8074, 390.379) radius 12
  circle A91 centre (154.1074, 390.379) radius 12
  circle A92 centre (187.4074, 390.379) radius 12
  circle A93 centre (220.7074, 390.379) radius 12
  circle A94 centre (254.0074, 390.379) radius 12
  circle A95 centre (287.3074, 390.379) radius 12
  circle A96 centre (320.6074, 390.379) radius 12
  circle A97 centre (353.9074, 390.379) radius 12
  circle A98 centre (387.2074, 390.379) radius 12
  circle A99 centre (420.5074, 390.379) radius 12
  circle A100 centre (87.5074, 428.379) radius 12
  circle A101 centre (120.8074, 428.379) radius 12
  circle A102 centre (154.1074, 428.379) radius 12
  circle A103 centre (187.4074, 428.379) radius 12
  circle A104 centre (220.7074, 428.379) radius 12
  circle A105 centre (254.0074, 428.379) radius 12
  circle A106 centre (287.3074, 428.379) radius 12
  circle A107 centre (320.6074, 428.379) radius 12
  circle A108 centre (353.9074, 428.379) radius 12
  circle A109 centre (387.2074, 428.379) radius 12
  circle A110 centre (420.5074, 428.379) radius 12
  circle A111 centre (28.1074, 490.979) radius 12
  circle A112 centre (479.9074, 490.979) radius 12
  circle A113 centre (287.3074, 352.379) radius 12
  line L8 (507.9074, 514.979) -> (0.1074, 514.979)
  line L9 (0.1074, 514.979) -> (0.1074, -0.221)
  line L10 (0.1074, -0.221) -> (507.9074, -0.221)
  line L11 (507.9074, -0.221) -> (507.9074, 514.979)
  line L12 (447.9074, 464.979) -> (497.9074, 464.979)
  line L13 (497.9074, 464.979) -> (497.9074, 49.779)
  line L14 (497.9074, 49.779) -> (447.9074, 49.779)
  line L15 (447.9074, 49.779) -> (447.9074, 464.979)
  dimension "d192" = 10
  dimension "d193" = 50
  dimension "d194" = 50
  dimension "d195" = 50
  constraint horizontal L12
  constraint vertical L13
  constraint horizontal L14
  constraint vertical L15
  measures "d192" distance of L11 L13
  measures "d193" distance of L13 L15
  measures "d194" distance of L8 L12
  measures "d195" distance of L10 L14
extrude "Extrusion5" cut sketch "Skizze6" against normal blind 20 contours L0 L7 L12 L13 L14 L15
sketch "Skizze7" plane through (0, 0, 0) normal (0, 0, -1) x (1, 0, 0)
  line L0 (447.9074, 49.779) -> (447.9074, 449.979)
  line L1 (447.9074, 449.979) -> (60.1074, 449.979)
  line L2 (60.1074, 449.979) -> (60.1074, 49.779)
  line L3 (60.1074, 49.779) -> (10.1074, 49.779)
  line L4 (10.1074, 49.779) -> (10.1074, 464.979)
  line L5 (10.1074, 464.979) -> (50.1074, 464.979)
  line L6 (50.1074, 464.979) -> (50.1074, 504.979)
  line L7 (50.1074, 504.979) -> (457.9074, 504.979)
  line L8 (457.9074, 504.979) -> (457.9074, 464.979)
  line L9 (457.9074, 464.979) -> (497.9074, 464.979)
  line L10 (497.9074, 464.979) -> (497.9074, 49.779)
  line L11 (497.9074, 49.779) -> (447.9074, 49.779)
  circle A0 centre (387.2074, 124.379) radius 12
  circle A1 centre (353.9074, 124.379) radius 12
  circle A2 centre (320.6074, 124.379) radius 12
  circle A3 centre (287.3074, 124.379) radius 12
  circle A4 centre (254.0074, 124.379) radius 12
  circle A5 centre (220.7074, 124.379) radius 12
  circle A6 centre (187.4074, 124.379) radius 12
  circle A7 centre (154.1074, 124.379) radius 12
  circle A8 centre (120.8074, 124.379) radius 12
  circle A9 centre (87.5074, 124.379) radius 12
  circle A10 centre (420.5074, 86.379) radius 12
  circle A11 centre (387.2074, 86.379) radius 12
  circle A12 centre (353.9074, 86.379) radius 12
  circle A13 centre (320.6074, 86.379) radius 12
  circle A14 centre (287.3074, 86.379) radius 12
  circle A15 centre (254.0074, 86.379) radius 12
  circle A16 centre (220.7074, 86.379) radius 12
  circle A17 centre (187.4074, 86.379) radius 12
  circle A18 centre (154.1074, 86.379) radius 12
  circle A19 centre (120.8074, 86.379) radius 12
  circle A20 centre (479.9074, 23.779) radius 12
  circle A21 centre (28.1074, 23.779) radius 10.8095
  circle A22 centre (87.5074, 86.379) radius 12
  circle A23 centre (387.2074, 238.379) radius 12
  circle A24 centre (420.5074, 238.379) radius 12
  circle A25 centre (87.5074, 276.379) radius 12
  circle A26 centre (120.8074, 276.379) radius 12
  circle A27 centre (154.1074, 276.379) radius 12
  circle A28 centre (187.4074, 276.379) radius 12
  circle A29 centre (220.7074, 276.379) radius 12
  circle A30 centre (254.0074, 276.379) radius 12
  circle A31 centre (287.3074, 276.379) radius 12
  circle A32 centre (320.6074, 276.379) radius 12
  circle A33 centre (353.9074, 276.379) radius 12
  circle A34 centre (387.2074, 276.379) radius 12
  circle A35 centre (420.5074, 276.379) radius 12
  circle A36 centre (87.5074, 314.379) radius 12
  circle A37 centre (120.8074, 314.379) radius 12
  circle A38 centre (154.1074, 314.379) radius 12
  circle A39 centre (187.4074, 314.379) radius 12
  circle A40 centre (220.7074, 314.379) radius 12
  circle A41 centre (254.0074, 314.379) radius 12
  circle A42 centre (287.3074, 314.379) radius 12
  circle A43 centre (320.6074, 314.379) radius 12
  circle A44 centre (353.9074, 314.379) radius 12
  circle A45 centre (387.2074, 314.379) radius 12
  circle A46 centre (420.5074, 314.379) radius 12
  circle A47 centre (87.5074, 352.379) radius 12
  circle A48 centre (120.8074, 352.379) radius 12
  circle A49 centre (154.1074, 352.379) radius 12
  circle A50 centre (187.4074, 352.379) radius 12
  circle A51 centre (220.7074, 352.379) radius 12
  circle A52 centre (254.0074, 352.379) radius 12
  circle A53 centre (353.9074, 238.379) radius 12
  circle A54 centre (320.6074, 238.379) radius 12
  circle A55 centre (287.3074, 238.379) radius 12
  circle A56 centre (254.0074, 238.379) radius 12
  circle A57 centre (220.7074, 238.379) radius 12
  circle A58 centre (187.4074, 238.379) radius 12
  circle A59 centre (154.1074, 238.379) radius 12
  circle A60 centre (120.8074, 238.379) radius 12
  circle A61 centre (87.5074, 238.379) radius 12
  circle A62 centre (420.5074, 200.379) radius 12
  circle A63 centre (387.2074, 200.379) radius 12
  circle A64 centre (353.9074, 200.379) radius 12
  circle A65 centre (320.6074, 200.379) radius 12
  circle A66 centre (287.3074, 200.379) radius 12
  circle A67 centre (254.0074, 200.379) radius 12
  circle A68 centre (220.7074, 200.379) radius 12
  circle A69 centre (187.4074, 200.379) radius 12
  circle A70 centre (154.1074, 200.379) radius 12
  circle A71 centre (120.8074, 200.379) radius 12
  circle A72 centre (87.5074, 200.379) radius 12
  circle A73 centre (420.5074, 162.379) radius 12
  circle A74 centre (387.2074, 162.379) radius 12
  circle A75 centre (353.9074, 162.379) radius 12
  circle A76 centre (320.6074, 162.379) radius 12
  circle A77 centre (287.3074, 162.379) radius 12
  circle A78 centre (254.0074, 162.379) radius 12
  circle A79 centre (220.7074, 162.379) radius 12
  circle A80 centre (187.4074, 162.379) radius 12
  circle A81 centre (154.1074, 162.379) radius 12
  circle A82 centre (120.8074, 162.379) radius 12
  circle A83 centre (87.5074, 162.379) radius 12
  circle A84 centre (420.5074, 124.379) radius 12
  circle A85 centre (320.6074, 352.379) radius 12
  circle A86 centre (353.9074, 352.379) radius 12
  circle A87 centre (387.2074, 352.379) radius 12
  circle A88 centre (420.5074, 352.379) radius 12
  circle A89 centre (87.5074, 390.379) radius 12
  circle A90 centre (120.8074, 390.379) radius 12
  circle A91 centre (154.1074, 390.379) radius 12
  circle A92 centre (187.4074, 390.379) radius 12
  circle A93 centre (220.7074, 390.379) radius 12
  circle A94 centre (254.0074, 390.379) radius 12
  circle A95 centre (287.3074, 390.379) radius 12
  circle A96 centre (320.6074, 390.379) radius 12
  circle A97 centre (353.9074, 390.379) radius 12
  circle A98 centre (387.2074, 390.379) radius 12
  circle A99 centre (420.5074, 390.379) radius 12
  circle A100 centre (87.5074, 428.379) radius 12
  circle A101 centre (120.8074, 428.379) radius 12
  circle A102 centre (154.1074, 428.379) radius 12
  circle A103 centre (187.4074, 428.379) radius 12
  circle A104 centre (220.7074, 428.379) radius 12
  circle A105 centre (254.0074, 428.379) radius 12
  circle A106 centre (287.3074, 428.379) radius 12
  circle A107 centre (320.6074, 428.379) radius 12
  circle A108 centre (353.9074, 428.379) radius 12
  circle A109 centre (387.2074, 428.379) radius 12
  circle A110 centre (420.5074, 428.379) radius 12
  circle A111 centre (28.1074, 490.979) radius 12
  circle A112 centre (479.9074, 490.979) radius 12
  circle A113 centre (287.3074, 352.379) radius 12
  line L12 (507.9074, 514.979) -> (0.1074, 514.979)
  line L13 (0.1074, 514.979) -> (0.1074, -0.221)
  line L14 (0.1074, -0.221) -> (507.9074, -0.221)
  line L15 (507.9074, -0.221) -> (507.9074, 514.979)
  line L16 (50.1074, 64.779) -> (457.9074, 64.779)
  line L17 (457.9074, 64.779) -> (457.9074, 9.779)
  line L18 (457.9074, 9.779) -> (50.1074, 9.779)
  line L19 (50.1074, 9.779) -> (50.1074, 64.779)
  dimension "d198" = 10
  dimension "d199" = 55
  dimension "d200" = 50
  dimension "d201" = 50
  constraint horizontal L16
  constraint vertical L17
  constraint horizontal L18
  constraint vertical L19
  measures "d198" distance of L14 L18
  measures "d199" distance of L16 L18
  measures "d200" distance of L13 L19
  measures "d201" distance of L15 L17
extrude "Extrusion6" cut sketch "Skizze7" against normal blind 20 contours L0 L2 L3 L11 L16 L17 L18 L19
sketch "Skizze8" plane through (0, 0, 0) normal (0, 0, -1) x (1, 0, 0)
  line L0 (60.1074, 64.779) -> (447.9074, 64.779)
  line L1 (447.9074, 64.779) -> (447.9074, 449.979)
  line L2 (447.9074, 449.979) -> (60.1074, 449.979)
  line L3 (60.1074, 449.979) -> (60.1074, 64.779)
  circle A0 centre (387.2074, 124.379) radius 12
  circle A1 centre (353.9074, 124.379) radius 12
  circle A2 centre (320.6074, 124.379) radius 12
  circle A3 centre (287.3074, 124.379) radius 12
  circle A4 centre (254.0074, 124.379) radius 12
  circle A5 centre (220.7074, 124.379) radius 12
  circle A6 centre (187.4074, 124.379) radius 12
  circle A7 centre (154.1074, 124.379) radius 12
  circle A8 centre (120.8074, 124.379) radius 12
  circle A9 centre (87.5074, 124.379) radius 12
  circle A10 centre (420.5074, 86.379) radius 12
  circle A11 centre (387.2074, 86.379) radius 12
  circle A12 centre (353.9074, 86.379) radius 12
  circle A13 centre (320.6074, 86.379) radius 12
  circle A14 centre (287.3074, 86.379) radius 12
  circle A15 centre (254.0074, 86.379) radius 12
  circle A16 centre (220.7074, 86.379) radius 12
  circle A17 centre (187.4074, 86.379) radius 12
  circle A18 centre (154.1074, 86.379) radius 12
  circle A19 centre (120.8074, 86.379) radius 12
  circle A20 centre (87.5074, 86.379) radius 12
  circle A21 centre (387.2074, 238.379) radius 12
  circle A22 centre (420.5074, 238.379) radius 12
  circle A23 centre (87.5074, 276.379) radius 12
  circle A24 centre (120.8074, 276.379) radius 12
  circle A25 centre (154.1074, 276.379) radius 12
  circle A26 centre (187.4074, 276.379) radius 12
  circle A27 centre (220.7074, 276.379) radius 12
  circle A28 centre (254.0074, 276.379) radius 12
  circle A29 centre (287.3074, 276.379) radius 12
  circle A30 centre (320.6074, 276.379) radius 12
  circle A31 centre (353.9074, 276.379) radius 12
  circle A32 centre (387.2074, 276.379) radius 12
  circle A33 centre (420.5074, 276.379) radius 12
  circle A34 centre (87.5074, 314.379) radius 12
  circle A35 centre (120.8074, 314.379) radius 12
  circle A36 centre (154.1074, 314.379) radius 12
  circle A37 centre (187.4074, 314.379) radius 12
  circle A38 centre (220.7074, 314.379) radius 12
  circle A39 centre (254.0074, 314.379) radius 12
  circle A40 centre (287.3074, 314.379) radius 12
  circle A41 centre (320.6074, 314.379) radius 12
  circle A42 centre (353.9074, 314.379) radius 12
  circle A43 centre (387.2074, 314.379) radius 12
  circle A44 centre (420.5074, 314.379) radius 12
  circle A45 centre (87.5074, 352.379) radius 12
  circle A46 centre (120.8074, 352.379) radius 12
  circle A47 centre (154.1074, 352.379) radius 12
  circle A48 centre (187.4074, 352.379) radius 12
  circle A49 centre (220.7074, 352.379) radius 12
  circle A50 centre (254.0074, 352.379) radius 12
  circle A51 centre (353.9074, 238.379) radius 12
  circle A52 centre (320.6074, 238.379) radius 12
  circle A53 centre (287.3074, 238.379) radius 12
  circle A54 centre (254.0074, 238.379) radius 12
  circle A55 centre (220.7074, 238.379) radius 12
  circle A56 centre (187.4074, 238.379) radius 12
  circle A57 centre (154.1074, 238.379) radius 12
  circle A58 centre (120.8074, 238.379) radius 12
  circle A59 centre (87.5074, 238.379) radius 12
  circle A60 centre (420.5074, 200.379) radius 12
  circle A61 centre (387.2074, 200.379) radius 12
  circle A62 centre (353.9074, 200.379) radius 12
  circle A63 centre (320.6074, 200.379) radius 12
  circle A64 centre (287.3074, 200.379) radius 12
  circle A65 centre (254.0074, 200.379) radius 12
  circle A66 centre (220.7074, 200.379) radius 12
  circle A67 centre (187.4074, 200.379) radius 12
  circle A68 centre (154.1074, 200.379) radius 12
  circle A69 centre (120.8074, 200.379) radius 12
  circle A70 centre (87.5074, 200.379) radius 12
  circle A71 centre (420.5074, 162.379) radius 12
  circle A72 centre (387.2074, 162.379) radius 12
  circle A73 centre (353.9074, 162.379) radius 12
  circle A74 centre (320.6074, 162.379) radius 12
  circle A75 centre (287.3074, 162.379) radius 12
  circle A76 centre (254.0074, 162.379) radius 12
  circle A77 centre (220.7074, 162.379) radius 12
  circle A78 centre (187.4074, 162.379) radius 12
  circle A79 centre (154.1074, 162.379) radius 12
  circle A80 centre (120.8074, 162.379) radius 12
  circle A81 centre (87.5074, 162.379) radius 12
  circle A82 centre (420.5074, 124.379) radius 12
  circle A83 centre (320.6074, 352.379) radius 12
  circle A84 centre (353.9074, 352.379) radius 12
  circle A85 centre (387.2074, 352.379) radius 12
  circle A86 centre (420.5074, 352.379) radius 12
  circle A87 centre (87.5074, 390.379) radius 12
  circle A88 centre (120.8074, 390.379) radius 12
  circle A89 centre (154.1074, 390.379) radius 12
  circle A90 centre (187.4074, 390.379) radius 12
  circle A91 centre (220.7074, 390.379) radius 12
  circle A92 centre (254.0074, 390.379) radius 12
  circle A93 centre (287.3074, 390.379) radius 12
  circle A94 centre (320.6074, 390.379) radius 12
  circle A95 centre (353.9074, 390.379) radius 12
  circle A96 centre (387.2074, 390.379) radius 12
  circle A97 centre (420.5074, 390.379) radius 12
  circle A98 centre (87.5074, 428.379) radius 12
  circle A99 centre (120.8074, 428.379) radius 12
  circle A100 centre (154.1074, 428.379) radius 12
  circle A101 centre (187.4074, 428.379) radius 12
  circle A102 centre (220.7074, 428.379) radius 12
  circle A103 centre (254.0074, 428.379) radius 12
  circle A104 centre (287.3074, 428.379) radius 12
  circle A105 centre (320.6074, 428.379) radius 12
  circle A106 centre (353.9074, 428.379) radius 12
  circle A107 centre (387.2074, 428.379) radius 12
  circle A108 centre (420.5074, 428.379) radius 12
  circle A109 centre (287.3074, 352.379) radius 12
  line L4 (60.1074, 434.379) -> (447.9074, 434.379)
  line L5 (447.9074, 434.379) -> (447.9074, 422.379)
  line L6 (447.9074, 422.379) -> (60.1074, 422.379)
  line L7 (60.1074, 422.379) -> (60.1074, 434.379)
  dimension "d204" = 6
  dimension "d205" = 6
  constraint horizontal L4
  constraint vertical L5
  constraint horizontal L6
  constraint vertical L7
  constraint collinear L3 L7
  constraint collinear L1 L5
  measures "d204" distance of A98.centre L4
  measures "d205" distance of A98.centre L6
extrude "Extrusion7" cut sketch "Skizze8" against normal blind 1 contours L3 A98 L4 L6 L7 | L1 A108 L4 L5 L6 | A98 A99 L4 L6 | A107 A108 L4 L6 | A99 A100 L4 L6 | A106 A107 L4 L6 | A100 A101 L4 L6 | A105 A106 L4 L6 | A101 A102 L4 L6 | A104 A105 L4 L6 | A102 A103 L4 L6 | A103 A104 L4 L6